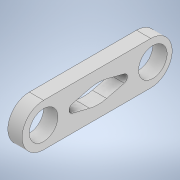
# Autodesk Inventor part: psmall
Saved by Autodesk Inventor 2022 (Build 260153000, 153)
## iProperties
Created: 2022-03-17
Part Number: psmall
Material: Generic
Document SubType Name: Modeling
Designer: br4ch
Density: 1 g/cm^3
Appearance: Default
Author: br4ch
Autodesk Inventor part; units mm, degrees
ref_plane "YZ Plane" through (0, 0, 0) normal (1, 0, 0) x (0, 1, 0)
ref_plane "XZ Plane" through (0, 0, 0) normal (0, 1, 0) x (-1, 0, 0)
ref_plane "XY Plane" through (0, 0, 0) normal (0, 0, 1) x (1, 0, 0)
sketch "Sketch1" plane through (0, 0, 0) normal (1, 0, 0) x (0, 1, 0)
  line L0 (0.5669, -17) -> (0.5669, -32) construction
  line L1 (-2.4331, -17) -> (-2.4331, -32)
  line L2 (3.5669, -32) -> (3.5669, -17)
  arc A0 (3.5669, -17) -> (-2.4331, -17) centre (0.5669, -17) ccw
  arc A1 (-2.4331, -32) -> (3.5669, -32) centre (0.5669, -32) ccw
  circle A2 centre (0.5669, -17) radius 2
  line L3 (-5.318, -24.6444) -> (5.6559, -24.6444) construction
  circle A3 centre (0.5669, -32.2888) radius 2
  line L4 (0.5669, -18.7744) -> (1.1337, -21) construction
  line L5 (0.5669, -30.5144) -> (1.1337, -28.2888) construction
  line L6 (0.5669, -18.7744) -> (0, -21) construction
  line L7 (0.5669, -30.5144) -> (0, -28.2888) construction
  arc A4 (1.1337, -21) -> (0, -21) centre (0.5669, -21.1444) ccw
  arc A5 (0, -28.2888) -> (1.1337, -28.2888) centre (0.5669, -28.1444) ccw
  arc A6 (1.7592, -25.8329) -> (1.7592, -23.4558) centre (-2.9073, -24.6444) ccw
  arc A7 (-0.6255, -23.4558) -> (-0.6255, -25.8329) centre (4.041, -24.6444) ccw
  line L8 (1.1337, -21) -> (1.7592, -23.4558)
  line L9 (0, -21) -> (-0.6255, -23.4558)
  line L10 (-0.6255, -25.8329) -> (-0.9282, -24.6444) construction
  line L11 (-0.6255, -23.4558) -> (-0.9282, -24.6444) construction
  line L12 (0, -28.2888) -> (-0.6255, -25.8329)
  line L13 (1.1337, -28.2888) -> (1.7592, -25.8329)
  line L14 (1.7592, -25.8329) -> (2.0619, -24.6444) construction
  line L15 (1.7592, -23.4558) -> (2.0619, -24.6444) construction
  point P0 (0, 0)
  point P1 (0.5669, -24.5)
  dimension "d0" = 6
  dimension "d1" = 15
  dimension "d2" = 4
  constraints: 34 end point, 16 tangent, 12 point on circle, 9 symmetric about line, 8 centre point, 4 point on line, 1 coincident, 1 horizontal, 1 midpoint, 1 parallel, 1 vertical, 3 other
  measures "d0" diameter of A1
  measures "d1" distance of L2.start L2.end
  measures "d2" diameter of A2
extrude "Extrusion1" add sketch "Sketch1" along normal blind 2
body "Solid1"
